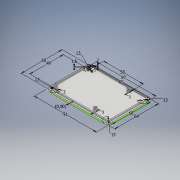
# Autodesk Inventor part: TapaIntermedia
Saved by Autodesk Inventor 2017 (Build 210142000, 142)
## iProperties
Part Number: TapaIntermedia
Material: Genérico
Document SubType Name: Modeling
Designer: danie
Density: 1 g/cm^3
Appearance: Valor por defecto
Author: danie
## iProperties of the stored document TapaIntermedia_3DPrint.ipt
Part Number: TapaIntermedia_3DPrint
Material: Genérico
Document SubType Name: Modeling
Designer: Daniel
Density: 1 g/cm^3
Appearance: Valor por defecto
Author: Daniel
Autodesk Inventor part; units mm, degrees
ref_plane "YZ Plane" through (0, 0, 0) normal (1, 0, 0) x (0, 1, 0)
ref_plane "XZ Plane" through (0, 0, 0) normal (0, 1, 0) x (-1, 0, 0)
ref_plane "XY Plane" through (0, 0, 0) normal (0, 0, 1) x (1, 0, 0)
sketch "Boceto1" plane through (0, 0, 0) normal (0, 0, 1) x (1, 0, 0)
  line L0 (-39, -32) -> (39, -32)
  line L1 (45.5, -25.5) -> (45.5, 25.5)
  line L2 (39, 32) -> (-39, 32)
  line L3 (-45.5, 25.5) -> (-45.5, -25.5)
  line L4 (-45.5, -32) -> (45.5, 32) construction
  line L5 (45.5, -32) -> (-45.5, 32) construction
  line L6 (-45.5, -32) -> (45.5, -32) construction
  arc A0 (-39, 32) -> (-45.5, 25.5) centre (-39, 25.5) ccw
  arc A1 (-45.5, -25.5) -> (-39, -32) centre (-39, -25.5) ccw
  arc A2 (45.5, 25.5) -> (39, 32) centre (39, 25.5) ccw
  arc A3 (39, -32) -> (45.5, -25.5) centre (39, -25.5) ccw
  line L7 (-43.5, 25.5) -> (-43.5, -25.5)
  arc A4 (-43.5, -25.5) -> (-39, -30) centre (-39, -25.5) ccw
  line L8 (-39, -30) -> (39, -30)
  arc A5 (39, -30) -> (43.5, -25.5) centre (39, -25.5) ccw
  line L9 (43.5, -25.5) -> (43.5, 25.5)
  arc A6 (43.5, 25.5) -> (39, 30) centre (39, 25.5) ccw
  line L10 (39, 30) -> (-39, 30)
  arc A7 (-39, 30) -> (-43.5, 25.5) centre (-39, 25.5) ccw
  line L11 (-42, 25.5) -> (-42, -25.5)
  arc A8 (-42, -25.5) -> (-39, -28.5) centre (-39, -25.5) ccw
  line L12 (-39, -28.5) -> (39, -28.5)
  arc A9 (39, -28.5) -> (42, -25.5) centre (39, -25.5) ccw
  line L13 (42, -25.5) -> (42, 25.5)
  arc A10 (42, 25.5) -> (39, 28.5) centre (39, 25.5) ccw
  line L14 (39, 28.5) -> (-39, 28.5)
  arc A11 (-39, 28.5) -> (-42, 25.5) centre (-39, 25.5) ccw
  circle A12 centre (-39, 24.5) radius 1.5
  circle A13 centre (-39, -24.5) radius 1.5
  circle A14 centre (19, 24.5) radius 1.5
  circle A15 centre (19, -24.5) radius 1.5
  line L15 (-42.5, 28) -> (42.5, 28) construction
  line L16 (42.5, 28) -> (42.5, -28) construction
  line L17 (42.5, -28) -> (-42.5, -28) construction
  line L18 (-42.5, -28) -> (-42.5, 28) construction
  line L19 (-42.5, 28) -> (42.5, -28) construction
  line L20 (42.5, 28) -> (-42.5, -28) construction
  point P0 (0, 0)
  dimension "d0" = 91
  dimension "d1" = 0
  dimension "d2" = 64
  dimension "d4" = 13
  dimension "d5" = 13
  dimension "d6" = 13
  dimension "d7" = 13
  dimension "d48" = 2
  dimension "d49" = 1.5
  dimension "d52" = 3
  dimension "d55" = 3
  dimension "d56" = 3
  dimension "d57" = 3
  dimension "d58" = 58
  dimension "d59" = 49
  dimension "d60" = 60
  dimension "d61" = 87
  dimension "d62" = 85
  dimension "d63" = 56
  dimension "d64" = 3.5
  dimension "d65" = 3.5
  constraints: 42 end point, 24 point on circle, 16 centre point, 8 parallel, 8 tangent, 4 midpoint, 4 perpendicular, 3 horizontal, 2 horizontal alignment, 2 point on line, 2 vertical alignment, 14 other
  measures "d0" distance of L4.start L5.start
  measures "d1" distance between parallel lines of L0 L6
  measures "d2" distance of L4.end L5.start
  measures "d4" diameter of A0
  measures "d5" diameter of A1
  measures "d6" diameter of A2
  measures "d7" diameter of A3
  measures "d48" radial gap between concentric circles of A0 A7
  measures "d49" radial gap between concentric circles of A7 A11
  measures "d52" diameter of A12
  measures "d55" diameter of A13
  measures "d56" diameter of A14
  measures "d57" diameter of A15
  measures "d58" distance of A14.centre A12.centre
  measures "d59" distance of A13.centre A12.centre
  measures "d60" distance between parallel lines of L8 L10
  measures "d61" distance between parallel lines of L9 L7
  measures "d62" distance of L15.start L15.end
  measures "d63" distance of L15.end L16.end
  measures "d64" distance from line of L15 A12.centre
  measures "d65" distance from line of L18 A12.centre
extrude "Extrusión3" add sketch "Boceto1" along normal mid plane 2.5 contours A1 L3 A0 L2 A2 L1 A3 L0 | A7 L10 A6 L9 A5 L8 A4 L7 | A11 L14 A10 L13 A9 L12 A8 L11
extrude "Extrusión4" add sketch "Boceto1" along normal mid plane 6 contours A7 L10 A6 L9 A5 L8 A4 L7
sketch "Boceto3" plane through (0, 0, 1.25) normal (0, 0, 1) x (1, 0, 0)
  arc A0 (-39, 28.5) -> (-42, 25.5) centre (-39, 25.5) ccw projected
  line L0 (-42, 25.5) -> (-42, -25.5) projected
  arc A1 (-42, -25.5) -> (-39, -28.5) centre (-39, -25.5) ccw projected
  line L1 (-39, -28.5) -> (39, -28.5) projected
  arc A2 (39, -28.5) -> (42, -25.5) centre (39, -25.5) ccw projected
  line L2 (42, -25.5) -> (42, 25.5) projected
  arc A3 (42, 25.5) -> (39, 28.5) centre (39, 25.5) ccw projected
  line L3 (39, 28.5) -> (-39, 28.5) projected
  circle A4 centre (19, -24.5) radius 1.5 projected
  circle A5 centre (19, 24.5) radius 1.5 projected
  circle A6 centre (-39, -24.5) radius 1.5 projected
  circle A7 centre (-39, 24.5) radius 1.5 projected
  circle A8 centre (-39, -24.5) radius 2.5
  circle A9 centre (-39, 24.5) radius 2.5
  circle A10 centre (19, -24.5) radius 2.5
  circle A11 centre (19, 24.5) radius 2.5
  point P0 (0, 0)
  dimension "d70" = 1
  dimension "d71" = 1
  dimension "d72" = 1
  dimension "d73" = 1
  constraints: 4 centre point
  measures "d70" radial gap between concentric circles of A6 A8
  measures "d71" radial gap between concentric circles of A7 A9
  measures "d72" radial gap between concentric circles of A4 A10
  measures "d73" radial gap between concentric circles of A5 A11
extrude "Extrusión5" add sketch "Boceto3" along normal blind 4 contours A8 | A9 | A10 | A11
